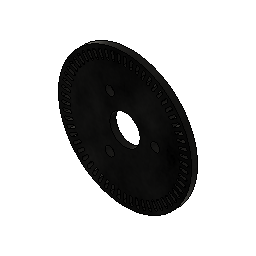
Encoder disc relative (Autodesk Fusion 360 design; units mm, degrees)
Autodesk Fusion 360 part; units mm, degrees
sketch "Sketch1" plane through (0, 0, 0) normal (0, 0, 1) x (1, 0, 0)
  arc A0 (20.0811, -3.7218) -> (19.8588, -4.7677) centre (19.9836, -4.2477) cw
  arc A1 (3.4027, 18.0763) -> (4.2438, 17.8975) centre (3.8318, 18.0274) ccw
  line L0 (9.7451, -17.9482) -> (8.822, -16.1401)
  arc A2 (4.7677, 19.8588) -> (3.7218, 20.0811) centre (4.2477, 19.9836) ccw
  arc A3 (19.2516, -6.8174) -> (19.5821, -5.8005) centre (19.4302, -6.3132) ccw
  arc A4 (8.7924, -18.4336) -> (7.8156, -18.8685) centre (8.3097, -18.6638) cw
  arc A5 (8.822, -16.1401) -> (9.5667, -15.7101) centre (9.215, -15.9609) cw
  arc A6 (18.2431, -2.3497) -> (18.3329, -1.4946) centre (18.3291, -1.9265) cw
  arc A7 (6.0913, -17.3559) -> (5.2735, -17.6216) centre (5.6952, -17.5281) ccw
  arc A8 (17.6216, -5.2735) -> (17.3559, -6.0913) centre (17.5281, -5.6952) ccw
  arc A9 (9.5667, -15.7101) -> (8.822, -16.1401) centre (9.215, -15.9609) ccw
  arc A10 (19.2516, -6.8174) -> (19.5821, -5.8005) centre (19.4302, -6.3132) ccw
  arc A11 (5.8005, -19.5821) -> (6.8174, -19.2516) centre (6.3132, -19.4302) ccw
  arc A12 (16.9738, -7.0866) -> (16.6241, -7.8721) centre (16.8367, -7.4962) ccw
  arc A13 (18.3329, -1.4946) -> (18.2431, -2.3497) centre (18.3291, -1.9265) ccw
  arc A14 (7.0866, -16.9738) -> (7.8721, -16.6241) centre (7.4962, -16.8367) cw
  arc A15 (10.671, -17.4135) -> (9.7451, -17.9482) centre (10.215, -17.693) cw
  line L1 (20.2484, -2.6657) -> (18.2431, -2.3497)
  line L2 (19.2516, -6.8174) -> (17.3559, -6.0913)
  arc A16 (11.1565, -14.6241) -> (10.4608, -15.1295) centre (10.8329, -14.9103) ccw
  line L3 (18.3329, -1.4946) -> (20.3601, -1.6024)
  arc A17 (11.1565, -14.6241) -> (10.4608, -15.1295) centre (10.8329, -14.9103) ccw
  arc A18 (7.8156, -18.8685) -> (8.7924, -18.4336) centre (8.3097, -18.6638) ccw
  line L4 (19.5821, -5.8005) -> (17.6216, -5.2735)
  arc A19 (5.2735, -17.6216) -> (6.0913, -17.3559) centre (5.6952, -17.5281) cw
  line L5 (17.6216, -5.2735) -> (19.5821, -5.8005)
  line L6 (16.9738, -7.0866) -> (18.8685, -7.8156)
  arc A20 (7.8721, -16.6241) -> (7.0866, -16.9738) centre (7.4962, -16.8367) ccw
  line L7 (19.8588, -4.7677) -> (17.8975, -4.2438)
  arc A21 (9.7451, -17.9482) -> (10.671, -17.4135) centre (10.215, -17.693) ccw
  line L8 (17.3559, -6.0913) -> (19.2516, -6.8174)
  arc A22 (6.8174, -19.2516) -> (5.8005, -19.5821) centre (6.3132, -19.4302) cw
  line L9 (18.0763, -3.4027) -> (20.0811, -3.7218)
  line L10 (19.8588, -4.7677) -> (17.8975, -4.2438)
  line L11 (16.9738, -7.0866) -> (18.8685, -7.8156)
  line L12 (18.3329, -1.4946) -> (20.3601, -1.6024)
  line L13 (20.2484, -2.6657) -> (18.2431, -2.3497)
  line L14 (18.0763, -3.4027) -> (20.0811, -3.7218)
  arc A23 (0.4299, 18.3887) -> (-0.4299, 18.3887) centre (0, 18.4301) cw
  arc A24 (-0.5346, 20.4161) -> (0.5346, 20.4161) centre (0, 20.4301) cw
  arc A25 (-3.7218, 20.0811) -> (-4.7677, 19.8588) centre (-4.2477, 19.9836) ccw
  arc A26 (-2.3497, 18.2431) -> (-1.4946, 18.333) centre (-1.9265, 18.3291) ccw
  arc A27 (-3.7218, 20.0811) -> (-4.7677, 19.8588) centre (-4.2477, 19.9836) ccw
  arc A28 (-4.2438, 17.8975) -> (-3.4027, 18.0763) centre (-3.8318, 18.0274) ccw
  arc A29 (-4.2438, 17.8975) -> (-3.4027, 18.0763) centre (-3.8318, 18.0274) ccw
  arc A30 (17.8975, 4.2438) -> (18.0763, 3.4027) centre (18.0273, 3.8318) ccw
  line L15 (-2.3497, -18.2431) -> (-2.6658, -20.2484)
  arc A31 (20.3601, 1.6024) -> (20.2484, 2.6658) centre (20.3182, 2.1355) ccw
  line L16 (0.4299, -18.3887) -> (0.5346, -20.4161)
  arc A32 (20.3601, 1.6024) -> (20.2484, 2.6658) centre (20.3182, 2.1355) ccw
  line L17 (2.3497, -18.2431) -> (2.6657, -20.2484)
  arc A33 (20.0811, 3.7218) -> (19.8588, 4.7677) centre (19.9836, 4.2477) ccw
  line L18 (-2.3497, -18.2431) -> (-2.6658, -20.2484)
  arc A34 (17.3559, 6.0913) -> (17.6216, 5.2735) centre (17.5281, 5.6952) ccw
  line L19 (-0.5346, -20.4161) -> (-0.4299, -18.3887)
  arc A35 (17.8975, 4.2438) -> (18.0763, 3.4027) centre (18.0273, 3.8318) ccw
  line L20 (1.4946, -18.3329) -> (1.6024, -20.3601)
  arc A36 (19.5821, 5.8005) -> (19.2516, 6.8174) centre (19.4302, 6.3132) ccw
  arc A37 (2.3497, -18.2431) -> (1.4946, -18.3329) centre (1.9265, -18.3291) ccw
  arc A38 (18.3887, -0.4299) -> (18.3887, 0.4299) centre (18.4301, 0) cw
  arc A39 (-0.5346, -20.4161) -> (0.5346, -20.4161) centre (0, -20.4301) ccw
  arc A40 (20.4161, -0.5346) -> (20.4161, 0.5346) centre (20.4301, 0) ccw
  arc A41 (2.3497, -18.2431) -> (1.4946, -18.3329) centre (1.9265, -18.3291) ccw
  arc A42 (18.2431, 2.3497) -> (18.3329, 1.4946) centre (18.3291, 1.9265) ccw
  arc A43 (-2.6658, -20.2484) -> (-1.6024, -20.3601) centre (-2.1355, -20.3182) ccw
  arc A44 (20.0811, 3.7218) -> (19.8588, 4.7677) centre (19.9836, 4.2477) ccw
  arc A45 (4.2438, -17.8975) -> (3.4027, -18.0763) centre (3.8318, -18.0273) ccw
  arc A46 (20.4161, 0.5346) -> (20.4161, -0.5346) centre (20.4301, 0) cw
  arc A47 (-2.6658, -20.2484) -> (-1.6024, -20.3601) centre (-2.1355, -20.3182) ccw
  line L21 (18.3329, 1.4946) -> (20.3601, 1.6024)
  arc A48 (-1.4946, -18.3329) -> (-2.3497, -18.2431) centre (-1.9265, -18.3291) ccw
  line L22 (19.8588, 4.7677) -> (17.8975, 4.2438)
  arc A49 (1.6024, -20.3601) -> (2.6657, -20.2484) centre (2.1355, -20.3182) ccw
  arc A50 (-1.4946, -18.3329) -> (-2.3497, -18.2431) centre (-1.9265, -18.3291) ccw
  arc A51 (-9.5667, 15.7101) -> (-8.822, 16.1401) centre (-9.215, 15.9609) ccw
  line L23 (17.6216, 5.2735) -> (19.5821, 5.8005)
  line L24 (17.3559, 6.0913) -> (19.2516, 6.8174)
  line L25 (-7.0866, 16.9738) -> (-7.8156, 18.8685)
  line L26 (-7.8722, 16.6241) -> (-8.7924, 18.4336)
  line L27 (-8.7924, 18.4336) -> (-7.8722, 16.6241)
  line L28 (-7.8156, 18.8685) -> (-7.0866, 16.9738)
  line L29 (17.8975, 4.2438) -> (19.8588, 4.7677)
  line L30 (-6.8174, 19.2517) -> (-6.0913, 17.3559)
  line L31 (-5.2735, 17.6216) -> (-5.8005, 19.5821)
  line L32 (-3.7218, -20.0811) -> (-3.4027, -18.0763)
  line L33 (-4.2438, -17.8975) -> (-4.7677, -19.8588)
  line L34 (-7.0866, -16.9738) -> (-7.8156, -18.8685)
  line L35 (-7.8156, -18.8685) -> (-7.0866, -16.9738)
  line L36 (-7.8722, -16.6241) -> (-8.7924, -18.4336)
  arc A52 (15.7101, 9.5667) -> (16.1401, 8.822) centre (15.9609, 9.215) ccw
  line L37 (-5.8005, -19.5821) -> (-5.2735, -17.6216)
  arc A53 (15.5298, 13.2637) -> (14.8144, 14.0583) centre (15.1825, 13.6704) ccw
  line L38 (-8.822, -16.1401) -> (-9.7451, -17.9482)
  arc A54 (16.6241, 7.8722) -> (16.9738, 7.0866) centre (16.8367, 7.4962) ccw
  line L39 (-6.0913, -17.3559) -> (-6.8174, -19.2516)
  arc A55 (18.8685, 7.8156) -> (18.4336, 8.7924) centre (18.6638, 8.3097) ccw
  line L40 (-6.0913, -17.3559) -> (-6.8174, -19.2516)
  arc A56 (14.0583, 14.8144) -> (13.2637, 15.5298) centre (13.6704, 15.1825) ccw
  arc A57 (11.985, 13.9532) -> (12.624, 13.3778) centre (12.3321, 13.6962) ccw
  line L41 (-8.7924, -18.4336) -> (-7.8722, -16.6241)
  arc A58 (13.3778, 12.624) -> (13.9532, 11.985) centre (13.6962, 12.3321) ccw
  line L42 (-3.4027, -18.0763) -> (-3.7218, -20.0811)
  arc A59 (18.8685, 7.8156) -> (18.4336, 8.7924) centre (18.6638, 8.3097) ccw
  line L43 (-5.8005, -19.5821) -> (-5.2735, -17.6216)
  arc A60 (12.4328, 16.2027) -> (11.5678, 16.8312) centre (12.0085, 16.5283) ccw
  line L44 (-9.7451, -17.9482) -> (-8.822, -16.1401)
  line L45 (-19.5821, -5.8005) -> (-17.6216, -5.2735)
  line L46 (-20.0811, -3.7218) -> (-18.0763, -3.4027)
  arc A61 (-13.3778, -12.624) -> (-13.9532, -11.985) centre (-13.6962, -12.3321) ccw
  line L47 (-20.4161, 0.5346) -> (-18.3887, 0.4299)
  arc A62 (-14.0583, -14.8144) -> (-13.2637, -15.5298) centre (-13.6704, -15.1825) ccw
  line L48 (-18.3887, -0.4299) -> (-20.4161, -0.5346)
  arc A63 (-10.671, -17.4135) -> (-9.7451, -17.9482) centre (-10.215, -17.693) ccw
  line L49 (-18.3887, 0.4299) -> (-20.4161, 0.5346)
  arc A64 (-12.4328, -16.2027) -> (-11.5678, -16.8312) centre (-12.0085, -16.5283) ccw
  line L50 (-19.8588, -4.7677) -> (-17.8975, -4.2438)
  arc A65 (-14.8144, -14.0583) -> (-15.5298, -13.2637) centre (-15.1825, -13.6704) cw
  line L51 (-18.333, -1.4946) -> (-20.3601, -1.6024)
  arc A66 (-13.9532, -11.985) -> (-13.3778, -12.624) centre (-13.6962, -12.3321) cw
  line L52 (-18.2431, 2.3497) -> (-20.2484, 2.6658)
  line L53 (-15.7101, 9.5667) -> (-17.4135, 10.671)
  line L54 (-20.2484, -2.6657) -> (-18.2431, -2.3497)
  line L55 (-20.3601, 1.6024) -> (-18.333, 1.4946)
  line L56 (-20.0811, 3.7218) -> (-18.0763, 3.4027)
  line L57 (-20.2484, 2.6658) -> (-18.2431, 2.3497)
  line L58 (-16.6241, 7.8722) -> (-18.4336, 8.7924)
  arc A67 (-20.4161, 0.5346) -> (-20.4161, -0.5346) centre (-20.4301, 0) ccw
  line L59 (-19.8588, 4.7677) -> (-17.8975, 4.2438)
  line L60 (-20.4161, -0.5346) -> (-18.3887, -0.4299)
  line L61 (-18.8685, 7.8156) -> (-16.9738, 7.0866)
  line L62 (-18.0763, -3.4027) -> (-20.0811, -3.7218)
  line L63 (-17.9482, 9.7451) -> (-16.1401, 8.822)
  line L64 (-20.3601, 1.6024) -> (-18.333, 1.4946)
  line L65 (-17.8975, 4.2438) -> (-19.8588, 4.7677)
  line L66 (-17.8975, -4.2438) -> (-19.8588, -4.7677)
  line L67 (-18.0763, 3.4027) -> (-20.0811, 3.7218)
  arc A68 (-1.6024, 20.3601) -> (-2.6658, 20.2484) centre (-2.1355, 20.3182) ccw
  arc A69 (-1.6024, 20.3601) -> (-2.6658, 20.2484) centre (-2.1355, 20.3182) ccw
  arc A70 (-2.3497, 18.2431) -> (-1.4946, 18.333) centre (-1.9265, 18.3291) ccw
  arc A71 (-0.4299, 18.3887) -> (0.4299, 18.3887) centre (0, 18.4301) ccw
  arc A72 (0.5346, 20.4161) -> (-0.5346, 20.4161) centre (0, 20.4301) ccw
  line L68 (-3.7218, 20.0811) -> (-3.4027, 18.0763)
  line L69 (-2.3497, 18.2431) -> (-2.6658, 20.2484)
  line L70 (-4.7677, 19.8588) -> (-4.2438, 17.8975)
  line L71 (-0.4299, 18.3887) -> (-0.5346, 20.4161)
  line L72 (0.5346, 20.4161) -> (0.4299, 18.3887)
  line L73 (-4.2438, 17.8975) -> (-4.7677, 19.8588)
  line L74 (-3.4027, 18.0763) -> (-3.7218, 20.0811)
  line L75 (-1.6024, 20.3601) -> (-1.4946, 18.333)
  line L76 (0.5346, -20.4161) -> (0.4299, -18.3887)
  line L77 (-2.6658, 20.2484) -> (-2.3497, 18.2431)
  line L78 (-0.4299, -18.3887) -> (-0.5346, -20.4161)
  line L79 (-1.4946, 18.333) -> (-1.6024, 20.3601)
  line L80 (3.7218, -20.0811) -> (3.4027, -18.0763)
  line L81 (0.5346, 20.4161) -> (0.4299, 18.3887)
  line L82 (4.7677, -19.8588) -> (4.2438, -17.8975)
  line L83 (-0.4299, 18.3887) -> (-0.5346, 20.4161)
  line L84 (-1.6024, -20.3601) -> (-1.4946, -18.3329)
  line L85 (1.6024, -20.3601) -> (1.4946, -18.3329)
  line L86 (-1.4946, -18.3329) -> (-1.6024, -20.3601)
  arc A73 (18.2431, 2.3497) -> (18.3329, 1.4946) centre (18.3291, 1.9265) ccw
  line L87 (4.2438, -17.8975) -> (4.7677, -19.8588)
  arc A74 (19.5821, 5.8005) -> (19.2516, 6.8174) centre (19.4302, 6.3132) ccw
  line L88 (3.4027, -18.0763) -> (3.7218, -20.0811)
  arc A75 (18.3887, 0.4299) -> (18.3887, -0.4299) centre (18.4301, 0) ccw
  line L89 (2.6657, -20.2484) -> (2.3497, -18.2431)
  arc A76 (17.3559, 6.0913) -> (17.6216, 5.2735) centre (17.5281, 5.6952) ccw
  line L90 (-11.985, 13.9532) -> (-13.2637, 15.5298)
  arc A77 (-13.3778, 12.624) -> (-13.9532, 11.985) centre (-13.6962, 12.3321) cw
  line L91 (-12.624, 13.3778) -> (-14.0583, 14.8144)
  line L92 (-12.4328, 16.2027) -> (-11.1565, 14.6241)
  line L93 (-11.5678, 16.8312) -> (-10.4608, 15.1295)
  arc A78 (-16.2027, 12.4328) -> (-16.8312, 11.5678) centre (-16.5283, 12.0085) ccw
  line L94 (-13.9532, 11.985) -> (-15.5298, 13.2637)
  line L95 (-10.4608, 15.1295) -> (-11.5678, 16.8312)
  arc A79 (-14.0583, 14.8144) -> (-13.2637, 15.5298) centre (-13.6704, 15.1825) cw
  arc A80 (-9.7451, 17.9482) -> (-10.671, 17.4135) centre (-10.215, 17.693) ccw
  line L96 (-12.624, 13.3778) -> (-14.0583, 14.8144)
  arc A81 (-16.2027, 12.4328) -> (-16.8312, 11.5678) centre (-16.5283, 12.0085) ccw
  line L97 (-11.1565, 14.6241) -> (-12.4328, 16.2027)
  arc A82 (-11.985, 13.9532) -> (-12.624, 13.3778) centre (-12.3321, 13.6962) cw
  line L98 (-13.2637, 15.5298) -> (-11.985, 13.9532)
  arc A83 (-11.5678, 16.8312) -> (-12.4328, 16.2027) centre (-12.0085, 16.5283) ccw
  line L99 (-14.6241, 11.1565) -> (-16.2027, 12.4328)
  line L100 (-9.5667, 15.7101) -> (-10.671, 17.4135)
  line L101 (-16.2027, 12.4328) -> (-14.6241, 11.1565)
  line L102 (-14.8144, 14.0583) -> (-13.3778, 12.624)
  arc A84 (-6.8174, -19.2516) -> (-5.8005, -19.5821) centre (-6.3132, -19.4302) ccw
  line L103 (15.1295, 10.4608) -> (16.8312, 11.5678)
  line L104 (-19.5821, -5.8005) -> (-17.6216, -5.2735)
  arc A85 (-6.8174, -19.2516) -> (-5.8005, -19.5821) centre (-6.3132, -19.4302) ccw
  line L105 (11.1565, 14.6241) -> (12.4328, 16.2027)
  line L106 (-16.9738, -7.0866) -> (-18.8685, -7.8156)
  arc A86 (-4.7677, -19.8588) -> (-3.7218, -20.0811) centre (-4.2477, -19.9836) ccw
  line L107 (14.8144, 14.0583) -> (13.3778, 12.624)
  arc A87 (-4.7677, -19.8588) -> (-3.7218, -20.0811) centre (-4.2477, -19.9836) ccw
  arc A88 (-14.6241, -11.1565) -> (-15.1295, -10.4608) centre (-14.9103, -10.8329) ccw
  line L108 (13.2637, 15.5298) -> (11.985, 13.9532)
  arc A89 (-3.4027, -18.0763) -> (-4.2438, -17.8975) centre (-3.8318, -18.0273) ccw
  arc A90 (-16.6241, -7.8721) -> (-16.9738, -7.0866) centre (-16.8367, -7.4962) ccw
  line L109 (18.8685, 7.8156) -> (16.9738, 7.0866)
  arc A91 (-15.7101, -9.5667) -> (-16.1401, -8.822) centre (-15.9609, -9.215) ccw
  arc A92 (-17.6216, -5.2735) -> (-17.3559, -6.0913) centre (-17.5281, -5.6952) cw
  arc A93 (-19.2517, -6.8174) -> (-19.5821, -5.8005) centre (-19.4302, -6.3132) cw
  arc A94 (-14.6241, -11.1565) -> (-15.1295, -10.4608) centre (-14.9103, -10.8329) ccw
  arc A95 (-18.8685, -7.8156) -> (-18.4336, -8.7924) centre (-18.6638, -8.3097) ccw
  arc A96 (-17.9482, -9.7451) -> (-17.4135, -10.671) centre (-17.693, -10.215) ccw
  arc A97 (-16.1401, -8.822) -> (-15.7101, -9.5667) centre (-15.9609, -9.215) cw
  arc A98 (13.2637, -15.5298) -> (14.0583, -14.8144) centre (13.6704, -15.1825) ccw
  arc A99 (-19.5821, -5.8005) -> (-19.2517, -6.8174) centre (-19.4302, -6.3132) ccw
  arc A100 (11.5678, -16.8312) -> (12.4328, -16.2027) centre (12.0085, -16.5283) ccw
  arc A101 (-16.6241, -7.8721) -> (-16.9738, -7.0866) centre (-16.8367, -7.4962) ccw
  arc A102 (13.2637, -15.5298) -> (14.0583, -14.8144) centre (13.6704, -15.1825) ccw
  arc A103 (-17.3559, -6.0913) -> (-17.6216, -5.2735) centre (-17.5281, -5.6952) ccw
  arc A104 (11.5678, -16.8312) -> (12.4328, -16.2027) centre (12.0085, -16.5283) ccw
  line L110 (11.985, -13.9532) -> (13.2637, -15.5298)
  line L111 (12.4328, -16.2027) -> (11.1565, -14.6241)
  arc A105 (-17.4135, -10.671) -> (-17.9482, -9.7451) centre (-17.693, -10.215) cw
  arc A106 (-18.333, 1.4946) -> (-18.2431, 2.3497) centre (-18.3291, 1.9265) ccw
  line L112 (-17.3559, 6.0913) -> (-19.2517, 6.8174)
  arc A107 (-18.2431, -2.3497) -> (-18.333, -1.4946) centre (-18.3291, -1.9265) ccw
  line L113 (-16.9738, 7.0866) -> (-18.8685, 7.8156)
  arc A108 (-18.3887, -0.4299) -> (-18.3887, 0.4299) centre (-18.4301, 0) ccw
  line L114 (-17.4135, 10.671) -> (-15.7101, 9.5667)
  arc A109 (-20.2484, 2.6658) -> (-20.3601, 1.6024) centre (-20.3182, 2.1355) ccw
  arc A110 (-18.333, 1.4946) -> (-18.2431, 2.3497) centre (-18.3291, 1.9265) ccw
  line L115 (-17.3559, 6.0913) -> (-19.2517, 6.8174)
  arc A111 (-20.0811, -3.7218) -> (-19.8588, -4.7677) centre (-19.9836, -4.2477) ccw
  line L116 (-15.1295, 10.4608) -> (-16.8312, 11.5678)
  arc A112 (-20.3601, -1.6024) -> (-20.2484, -2.6657) centre (-20.3182, -2.1355) ccw
  line L117 (-18.4336, 8.7924) -> (-16.6241, 7.8722)
  arc A113 (-20.4161, 0.5346) -> (-20.4161, -0.5346) centre (-20.4301, 0) ccw
  line L118 (-16.1401, 8.822) -> (-17.9482, 9.7451)
  arc A114 (-20.2484, 2.6658) -> (-20.3601, 1.6024) centre (-20.3182, 2.1355) ccw
  line L119 (-19.5821, 5.8005) -> (-17.6216, 5.2735)
  arc A115 (-17.8975, -4.2438) -> (-18.0763, -3.4027) centre (-18.0274, -3.8318) ccw
  line L120 (-19.5821, 5.8005) -> (-17.6216, 5.2735)
  arc A116 (-17.8975, -4.2438) -> (-18.0763, -3.4027) centre (-18.0274, -3.8318) ccw
  line L121 (-16.8312, 11.5678) -> (-15.1295, 10.4608)
  arc A117 (-20.3601, -1.6024) -> (-20.2484, -2.6657) centre (-20.3182, -2.1355) ccw
  arc A118 (-19.2517, 6.8174) -> (-19.5821, 5.8005) centre (-19.4302, 6.3132) ccw
  arc A119 (-20.0811, -3.7218) -> (-19.8588, -4.7677) centre (-19.9836, -4.2477) ccw
  arc A120 (-15.1295, 10.4608) -> (-14.6241, 11.1565) centre (-14.9103, 10.8329) ccw
  arc A121 (-18.3887, -0.4299) -> (-18.3887, 0.4299) centre (-18.4301, 0) ccw
  arc A122 (-19.8588, 4.7677) -> (-20.0811, 3.7218) centre (-19.9836, 4.2477) ccw
  arc A123 (-18.2431, -2.3497) -> (-18.333, -1.4946) centre (-18.3291, -1.9265) ccw
  arc A124 (-17.6216, 5.2735) -> (-17.3559, 6.0913) centre (-17.5281, 5.6952) ccw
  arc A125 (-19.2517, 6.8174) -> (-19.5821, 5.8005) centre (-19.4302, 6.3132) ccw
  arc A126 (-16.1401, 8.822) -> (-15.7101, 9.5667) centre (-15.9609, 9.215) ccw
  arc A127 (-9.7451, 17.9482) -> (-10.671, 17.4135) centre (-10.215, 17.693) ccw
  arc A128 (-16.9738, 7.0866) -> (-16.6241, 7.8722) centre (-16.8367, 7.4962) ccw
  arc A129 (-18.4336, 8.7924) -> (-18.8685, 7.8156) centre (-18.6638, 8.3097) ccw
  arc A130 (-17.4135, 10.671) -> (-17.9482, 9.7451) centre (-17.693, 10.215) ccw
  arc A131 (-17.4135, 10.671) -> (-17.9482, 9.7451) centre (-17.693, 10.215) ccw
  arc A132 (-17.6216, 5.2735) -> (-17.3559, 6.0913) centre (-17.5281, 5.6952) ccw
  arc A133 (-11.5678, 16.8312) -> (-12.4328, 16.2027) centre (-12.0085, 16.5283) ccw
  arc A134 (-15.1295, 10.4608) -> (-14.6241, 11.1565) centre (-14.9103, 10.8329) ccw
  arc A135 (-18.4336, 8.7924) -> (-18.8685, 7.8156) centre (-18.6638, 8.3097) ccw
  arc A136 (-18.0763, 3.4027) -> (-17.8975, 4.2438) centre (-18.0274, 3.8318) ccw
  arc A137 (-18.0763, 3.4027) -> (-17.8975, 4.2438) centre (-18.0274, 3.8318) ccw
  arc A138 (-15.5298, 13.2637) -> (-14.8144, 14.0583) centre (-15.1825, 13.6704) cw
  arc A139 (-16.9738, 7.0866) -> (-16.6241, 7.8722) centre (-16.8367, 7.4962) ccw
  arc A140 (-13.2637, 15.5298) -> (-14.0583, 14.8144) centre (-13.6704, 15.1825) ccw
  arc A141 (-19.8588, 4.7677) -> (-20.0811, 3.7218) centre (-19.9836, 4.2477) ccw
  arc A142 (-16.1401, 8.822) -> (-15.7101, 9.5667) centre (-15.9609, 9.215) ccw
  arc A143 (-12.624, 13.3778) -> (-11.985, 13.9532) centre (-12.3321, 13.6962) ccw
  arc A144 (-11.1565, 14.6241) -> (-10.4608, 15.1295) centre (-10.8329, 14.9103) ccw
  line L122 (-13.9532, 11.985) -> (-15.5298, 13.2637)
  arc A145 (-11.1565, 14.6241) -> (-10.4608, 15.1295) centre (-10.8329, 14.9103) ccw
  line L123 (-10.671, 17.4135) -> (-9.5667, 15.7101)
  arc A146 (-14.8144, 14.0583) -> (-15.5298, 13.2637) centre (-15.1825, 13.6704) ccw
  arc A147 (-13.9532, 11.985) -> (-13.3778, 12.624) centre (-13.6962, 12.3321) ccw
  line L124 (-14.8144, 14.0583) -> (-13.3778, 12.624)
  line L125 (13.3778, -12.624) -> (14.8144, -14.0583)
  circle A148 centre (0, 0) radius 22
  arc A149 (16.2027, -12.4328) -> (16.8312, -11.5678) centre (16.5283, -12.0085) ccw
  arc A150 (15.1295, -10.4608) -> (14.6241, -11.1565) centre (14.9103, -10.8329) ccw
  arc A151 (12.624, -13.3778) -> (11.985, -13.9532) centre (12.3321, -13.6962) ccw
  arc A152 (14.6241, -11.1565) -> (15.1295, -10.4608) centre (14.9103, -10.8329) cw
  arc A153 (18.4336, -8.7924) -> (18.8685, -7.8156) centre (18.6638, -8.3097) ccw
  arc A154 (16.1401, -8.822) -> (15.7101, -9.5667) centre (15.9609, -9.215) ccw
  circle A155 centre (10, 0) radius 1.5
  arc A156 (16.8312, -11.5678) -> (16.2027, -12.4328) centre (16.5283, -12.0085) cw
  arc A157 (17.4135, -10.671) -> (17.9482, -9.7451) centre (17.693, -10.215) ccw
  circle A158 centre (0, 0) radius 5
  arc A159 (13.9532, -11.985) -> (13.3778, -12.624) centre (13.6962, -12.3321) ccw
  circle A160 centre (-5, 8.6603) radius 1.5
  arc A161 (16.1401, -8.822) -> (15.7101, -9.5667) centre (15.9609, -9.215) ccw
  arc A162 (3.7218, -20.0811) -> (4.7677, -19.8588) centre (4.2477, -19.9836) ccw
  arc A163 (-6.0913, 17.3559) -> (-5.2735, 17.6216) centre (-5.6952, 17.5281) ccw
  line L126 (18.3887, 0.4299) -> (20.4161, 0.5346)
  arc A164 (-7.8156, 18.8685) -> (-8.7924, 18.4336) centre (-8.3097, 18.6638) ccw
  arc A165 (3.7218, -20.0811) -> (4.7677, -19.8588) centre (4.2477, -19.9836) ccw
  line L127 (20.4161, -0.5346) -> (18.3887, -0.4299)
  arc A166 (-5.8005, 19.5821) -> (-6.8174, 19.2517) centre (-6.3132, 19.4302) ccw
  arc A167 (1.6024, -20.3601) -> (2.6657, -20.2484) centre (2.1355, -20.3182) ccw
  arc A168 (-7.8156, 18.8685) -> (-8.7924, 18.4336) centre (-8.3097, 18.6638) ccw
  line L128 (18.3887, 0.4299) -> (20.4161, 0.5346)
  arc A169 (0.4299, -18.3887) -> (-0.4299, -18.3887) centre (0, -18.4301) ccw
  line L129 (18.2431, 2.3497) -> (20.2484, 2.6658)
  arc A170 (4.2438, -17.8975) -> (3.4027, -18.0763) centre (3.8318, -18.0273) ccw
  line L130 (20.4161, -0.5346) -> (18.3887, -0.4299)
  arc A171 (-6.0913, 17.3559) -> (-5.2735, 17.6216) centre (-5.6952, 17.5281) ccw
  arc A172 (0.4299, -18.3887) -> (-0.4299, -18.3887) centre (0, -18.4301) ccw
  line L131 (19.2516, 6.8174) -> (17.3559, 6.0913)
  arc A173 (-5.8005, 19.5821) -> (-6.8174, 19.2517) centre (-6.3132, 19.4302) ccw
  line L132 (20.2484, 2.6658) -> (18.2431, 2.3497)
  arc A174 (-7.8722, 16.6241) -> (-7.0866, 16.9738) centre (-7.4962, 16.8367) ccw
  arc A175 (-0.5346, -20.4161) -> (0.5346, -20.4161) centre (0, -20.4301) ccw
  arc A176 (-9.5667, 15.7101) -> (-8.822, 16.1401) centre (-9.215, 15.9609) ccw
  line L133 (19.5821, 5.8005) -> (17.6216, 5.2735)
  arc A177 (-7.8722, 16.6241) -> (-7.0866, 16.9738) centre (-7.4962, 16.8367) ccw
  line L134 (18.0763, 3.4027) -> (20.0811, 3.7218)
  line L135 (-9.7451, 17.9482) -> (-8.822, 16.1401)
  line L136 (20.0811, 3.7218) -> (18.0763, 3.4027)
  line L137 (-6.0913, 17.3559) -> (-6.8174, 19.2517)
  line L138 (20.3601, 1.6024) -> (18.3329, 1.4946)
  line L139 (-8.822, 16.1401) -> (-9.7451, 17.9482)
  line L140 (-5.8005, 19.5821) -> (-5.2735, 17.6216)
  arc A178 (16.8312, 11.5678) -> (16.2027, 12.4328) centre (16.5283, 12.0085) ccw
  line L141 (-4.7677, -19.8588) -> (-4.2438, -17.8975)
  line L142 (-17.9482, -9.7451) -> (-16.1401, -8.822)
  arc A179 (14.6241, 11.1565) -> (15.1295, 10.4608) centre (14.9103, 10.8329) ccw
  arc A180 (-8.822, -16.1401) -> (-9.5667, -15.7101) centre (-9.215, -15.9609) ccw
  line L143 (-15.7101, -9.5667) -> (-17.4135, -10.671)
  arc A181 (-8.7924, -18.4336) -> (-7.8156, -18.8685) centre (-8.3097, -18.6638) ccw
  arc A182 (17.9482, 9.7451) -> (17.4135, 10.671) centre (17.693, 10.215) ccw
  line L144 (-17.9482, -9.7451) -> (-16.1401, -8.822)
  line L145 (16.2027, 12.4328) -> (14.6241, 11.1565)
  arc A183 (-8.822, -16.1401) -> (-9.5667, -15.7101) centre (-9.215, -15.9609) ccw
  line L146 (-18.8685, -7.8156) -> (-16.9738, -7.0866)
  arc A184 (-8.7924, -18.4336) -> (-7.8156, -18.8685) centre (-8.3097, -18.6638) ccw
  line L147 (-15.1295, -10.4608) -> (-16.8312, -11.5678)
  line L148 (16.1401, 8.822) -> (17.9482, 9.7451)
  line L149 (16.9738, 7.0866) -> (18.8685, 7.8156)
  arc A185 (-5.2735, -17.6216) -> (-6.0913, -17.3559) centre (-5.6952, -17.5281) ccw
  line L150 (-16.8312, -11.5678) -> (-15.1295, -10.4608)
  line L151 (12.624, 13.3778) -> (14.0583, 14.8144)
  arc A186 (-7.0866, -16.9738) -> (-7.8722, -16.6241) centre (-7.4962, -16.8367) ccw
  line L152 (-18.4336, -8.7924) -> (-16.6241, -7.8721)
  line L153 (17.4135, 10.671) -> (15.7101, 9.5667)
  arc A187 (-3.4027, -18.0763) -> (-4.2438, -17.8975) centre (-3.8318, -18.0273) ccw
  line L154 (-16.6241, -7.8721) -> (-18.4336, -8.7924)
  line L155 (-15.7101, -9.5667) -> (-17.4135, -10.671)
  line L156 (18.4336, 8.7924) -> (16.6241, 7.8722)
  arc A188 (-7.0866, -16.9738) -> (-7.8722, -16.6241) centre (-7.4962, -16.8367) ccw
  arc A189 (-5.2735, -17.6216) -> (-6.0913, -17.3559) centre (-5.6952, -17.5281) ccw
  line L157 (-17.3559, -6.0913) -> (-19.2517, -6.8174)
  line L158 (13.9532, 11.985) -> (15.5298, 13.2637)
  line L159 (-17.3559, -6.0913) -> (-19.2517, -6.8174)
  arc A190 (6.8174, 19.2517) -> (5.8005, 19.5821) centre (6.3132, 19.4302) ccw
  line L160 (5.8005, -19.5821) -> (5.2735, -17.6216)
  arc A191 (7.0866, 16.9738) -> (7.8721, 16.6241) centre (7.4962, 16.8367) ccw
  arc A192 (19.8588, -4.7677) -> (20.0811, -3.7218) centre (19.9836, -4.2477) ccw
  line L161 (9.5667, -15.7101) -> (10.671, -17.4135)
  arc A193 (3.4027, 18.0763) -> (4.2438, 17.8975) centre (3.8318, 18.0274) ccw
  line L162 (6.0913, -17.3559) -> (6.8174, -19.2516)
  arc A194 (4.7677, 19.8588) -> (3.7218, 20.0811) centre (4.2477, 19.9836) ccw
  arc A195 (20.2484, -2.6657) -> (20.3601, -1.6024) centre (20.3182, -2.1355) ccw
  arc A196 (5.2735, 17.6216) -> (6.0913, 17.3559) centre (5.6952, 17.5281) ccw
  line L163 (9.5667, -15.7101) -> (10.671, -17.4135)
  arc A197 (18.0763, -3.4027) -> (17.8975, -4.2438) centre (18.0273, -3.8318) ccw
  arc A198 (6.8174, 19.2517) -> (5.8005, 19.5821) centre (6.3132, 19.4302) ccw
  line L164 (7.8721, -16.6241) -> (8.7924, -18.4336)
  arc A199 (17.6216, -5.2735) -> (17.3559, -6.0913) centre (17.5281, -5.6952) ccw
  line L165 (7.8721, 16.6241) -> (8.7924, 18.4336)
  line L166 (9.7451, 17.9482) -> (8.822, 16.1401)
  line L167 (5.8005, 19.5821) -> (5.2735, 17.6216)
  line L168 (4.7677, 19.8588) -> (4.2438, 17.8975)
  line L169 (3.4027, 18.0763) -> (3.7218, 20.0811)
  line L170 (11.5678, 16.8312) -> (10.4608, 15.1295)
  line L171 (1.6024, 20.3601) -> (1.4946, 18.333)
  line L172 (6.0913, 17.3559) -> (6.8174, 19.2517)
  line L173 (2.3497, 18.2431) -> (2.6657, 20.2484)
  line L174 (9.5667, 15.7101) -> (10.671, 17.4135)
  line L175 (7.8156, 18.8685) -> (7.0866, 16.9738)
  line L176 (5.8005, 19.5821) -> (5.2735, 17.6216)
  line L177 (11.5678, -16.8312) -> (10.4608, -15.1295)
  arc A200 (8.822, 16.1401) -> (9.5667, 15.7101) centre (9.215, 15.9609) ccw
  line L178 (6.0913, -17.3559) -> (6.8174, -19.2516)
  arc A201 (-18.8685, -7.8156) -> (-18.4336, -8.7924) centre (-18.6638, -8.3097) ccw
  line L179 (13.2637, -15.5298) -> (11.985, -13.9532)
  line L180 (11.1565, -14.6241) -> (12.4328, -16.2027)
  line L181 (-15.5298, -13.2637) -> (-13.9532, -11.985)
  line L182 (-13.3778, -12.624) -> (-14.8144, -14.0583)
  line L183 (-11.985, -13.9532) -> (-13.2637, -15.5298)
  line L184 (-14.6241, -11.1565) -> (-16.2027, -12.4328)
  line L185 (-10.4608, -15.1295) -> (-11.5678, -16.8312)
  line L186 (-13.3778, -12.624) -> (-14.8144, -14.0583)
  line L187 (-12.624, -13.3778) -> (-14.0583, -14.8144)
  line L188 (-10.671, -17.4135) -> (-9.5667, -15.7101)
  line L189 (-11.5678, -16.8312) -> (-10.4608, -15.1295)
  line L190 (-11.985, -13.9532) -> (-13.2637, -15.5298)
  line L191 (-12.4328, -16.2027) -> (-11.1565, -14.6241)
  line L192 (-14.0583, -14.8144) -> (-12.624, -13.3778)
  line L193 (-9.5667, -15.7101) -> (-10.671, -17.4135)
  line L194 (-15.5298, -13.2637) -> (-13.9532, -11.985)
  line L195 (-11.1565, -14.6241) -> (-12.4328, -16.2027)
  line L196 (-16.2027, -12.4328) -> (-14.6241, -11.1565)
  arc A202 (-10.671, -17.4135) -> (-9.7451, -17.9482) centre (-10.215, -17.693) ccw
  arc A203 (-13.2637, -15.5298) -> (-14.0583, -14.8144) centre (-13.6704, -15.1825) cw
  arc A204 (-10.4608, -15.1295) -> (-11.1565, -14.6241) centre (-10.8329, -14.9103) ccw
  arc A205 (-16.8312, -11.5678) -> (-16.2027, -12.4328) centre (-16.5283, -12.0085) ccw
  arc A206 (-12.4328, -16.2027) -> (-11.5678, -16.8312) centre (-12.0085, -16.5283) ccw
  arc A207 (-16.8312, -11.5678) -> (-16.2027, -12.4328) centre (-16.5283, -12.0085) ccw
  arc A208 (-15.5298, -13.2637) -> (-14.8144, -14.0583) centre (-15.1825, -13.6704) ccw
  arc A209 (-11.985, -13.9532) -> (-12.624, -13.3778) centre (-12.3321, -13.6962) ccw
  line L197 (-20.3601, -1.6024) -> (-18.333, -1.4946)
  arc A210 (-10.4608, -15.1295) -> (-11.1565, -14.6241) centre (-10.8329, -14.9103) ccw
  line L198 (-18.2431, -2.3497) -> (-20.2484, -2.6657)
  arc A211 (-12.624, -13.3778) -> (-11.985, -13.9532) centre (-12.3321, -13.6962) cw
  arc A212 (10.671, 17.4135) -> (9.7451, 17.9482) centre (10.215, 17.693) ccw
  line L199 (7.8721, -16.6241) -> (8.7924, -18.4336)
  arc A213 (16.6241, -7.8721) -> (16.9738, -7.0866) centre (16.8367, -7.4962) cw
  arc A214 (1.4946, 18.333) -> (2.3497, 18.2431) centre (1.9265, 18.3291) ccw
  line L200 (7.0866, -16.9738) -> (7.8156, -18.8685)
  arc A215 (8.7924, 18.4336) -> (7.8156, 18.8685) centre (8.3097, 18.6638) ccw
  line L201 (9.7451, -17.9482) -> (8.822, -16.1401)
  arc A216 (2.6657, 20.2484) -> (1.6024, 20.3601) centre (2.1355, 20.3182) ccw
  line L202 (7.8156, -18.8685) -> (7.0866, -16.9738)
  arc A217 (2.6657, 20.2484) -> (1.6024, 20.3601) centre (2.1355, 20.3182) ccw
  arc A218 (20.3601, -1.6024) -> (20.2484, -2.6657) centre (20.3182, -2.1355) cw
  line L203 (10.4608, -15.1295) -> (11.5678, -16.8312)
  arc A219 (1.4946, 18.333) -> (2.3497, 18.2431) centre (1.9265, 18.3291) ccw
  arc A220 (17.8975, -4.2438) -> (18.0763, -3.4027) centre (18.0273, -3.8318) cw
  line L204 (5.8005, -19.5821) -> (5.2735, -17.6216)
  line L205 (16.2027, -12.4328) -> (14.6241, -11.1565)
  line L206 (18.4336, -8.7924) -> (16.6241, -7.8721)
  line L207 (14.0583, -14.8144) -> (12.624, -13.3778)
  line L208 (18.4336, -8.7924) -> (16.6241, -7.8721)
  line L209 (13.9532, -11.985) -> (15.5298, -13.2637)
  line L210 (15.1295, -10.4608) -> (16.8312, -11.5678)
  line L211 (15.5298, -13.2637) -> (13.9532, -11.985)
  line L212 (12.624, -13.3778) -> (14.0583, -14.8144)
  line L213 (16.2027, -12.4328) -> (14.6241, -11.1565)
  line L214 (17.9482, -9.7451) -> (16.1401, -8.822)
  line L215 (15.7101, -9.5667) -> (17.4135, -10.671)
  line L216 (3.7218, 20.0811) -> (3.4027, 18.0763)
  line L217 (4.2438, 17.8975) -> (4.7677, 19.8588)
  line L218 (2.6657, 20.2484) -> (2.3497, 18.2431)
  line L219 (1.4946, 18.333) -> (1.6024, 20.3601)
  line L220 (15.1295, -10.4608) -> (16.8312, -11.5678)
  line L221 (17.4135, -10.671) -> (15.7101, -9.5667)
  line L222 (14.8144, -14.0583) -> (13.3778, -12.624)
  line L223 (16.1401, -8.822) -> (17.9482, -9.7451)
  arc A221 (18.8685, -7.8156) -> (18.4336, -8.7924) centre (18.6638, -8.3097) cw
  arc A222 (13.9532, -11.985) -> (13.3778, -12.624) centre (13.6962, -12.3321) ccw
  arc A223 (14.8144, -14.0583) -> (15.5298, -13.2637) centre (15.1825, -13.6704) ccw
  arc A224 (17.4135, -10.671) -> (17.9482, -9.7451) centre (17.693, -10.215) ccw
  arc A225 (12.624, -13.3778) -> (11.985, -13.9532) centre (12.3321, -13.6962) ccw
  circle A226 centre (-5, -8.6603) radius 1.5
  arc A227 (10.4608, 15.1295) -> (11.1565, 14.6241) centre (10.8329, 14.9103) ccw
  arc A228 (14.8144, -14.0583) -> (15.5298, -13.2637) centre (15.1825, -13.6704) ccw
  dimension "d2654" = 0
  dimension "d2670" = 0
extrude "Extrude1" add sketch "Sketch1" along normal blind 2
